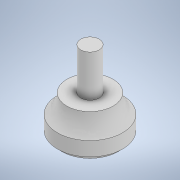
# Autodesk Inventor part: Ch7(5) Part 8 Rack Pad
Saved by Autodesk Inventor 2020 (Build 240168000, 168)
## iProperties
Created: 2021-03-04
Part Number: Ch7(5) Part 8 Rack Pad
Material: Generic
Document SubType Name: Modeling
Designer: adriggs
Density: 1 g/cm^3
Appearance: Default
Author: adriggs
Autodesk Inventor part; units mm, degrees
ref_plane "YZ Plane" through (0, 0, 0) normal (1, 0, 0) x (0, 1, 0)
ref_plane "XZ Plane" through (0, 0, 0) normal (0, 1, 0) x (-1, 0, 0)
ref_plane "XY Plane" through (0, 0, 0) normal (0, 0, 1) x (1, 0, 0)
sketch "Sketch1" plane through (0, 0, 0) normal (0, 0, 1) x (1, 0, 0)
  line L0 (0, -6.919) -> (0, 30.8458) projected
  line L1 (-3.175, 0) -> (19.05, 0) projected
  line L2 (0, 0) -> (11.1125, 0)
  line L3 (9.5885, -1.524) -> (11.1125, 0)
  line L4 (9.5885, -1.524) -> (0, -1.524)
  line L5 (11.1125, 0) -> (11.1125, 4.826)
  line L6 (0, 11.176) -> (7.9375, 11.176)
  line L7 (0, 25.4508) -> (3.175, 25.4508)
  line L8 (3.175, 25.4508) -> (3.175, 11.176)
  arc A0 (7.9375, 11.176) -> (11.1125, 4.826) centre (15.875, 11.176) ccw
  dimension "d9" = 11.1125
  dimension "d12" = 1.524
  dimension "d13" = 45
  dimension "d18" = 6.35
  dimension "d19" = 7.9375
  dimension "d20" = 12.7
  dimension "d22" = 3.175
  dimension "d23" = 26.9748
  constraints: 14 end point, 6 point on line, 3 perpendicular, 2 point on circle, 1 centre point, 1 horizontal, 1 vertical
  measures "d9" distance of L2.end L2.start
  measures "d12" distance between parallel lines of L4 L1
  measures "d13" angle of L4 L3
  measures "d18" vertical distance of L5.end L3.start
  measures "d19" distance of L6.start L6.end
  measures "d20" vertical distance of L6.end L3.start
  measures "d22" distance of L7.start L7.end
  measures "d23" vertical distance of L3.start L7.end
revolve "Revolution1" add sketch "Sketch1" angle 360 about axis through (0, -10, 0) along (0, 1, 0)
body "Solid1"
